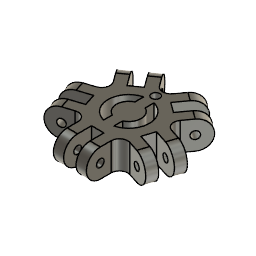
CenterRingV0_v10 (Autodesk Fusion 360 design; units mm, degrees)
Autodesk Fusion 360 part; units mm, degrees
sketch "Sketch1" plane through (0, 0, 0) normal (0, 0, 1) x (1, 0, 0)
  circle A0 centre (0, 0) radius 5
  circle A1 centre (0, 0) radius 7.5
  line L0 (0, 0) -> (0, -7.5) construction
  line L1 (0, -7.5) -> (1.5, -7.5) construction
  line L2 (0, -7.5) -> (-1.5, -7.5) construction
  line L3 (-1.5, -7.5) -> (-1.5, -7.3485)
  line L4 (1.5, -7.5) -> (1.5, -7.3485)
  line L5 (1.5, -7.5) -> (1.5, -14.25)
  line L6 (0, -7.5) -> (0, -9.25) construction
  line L7 (0, -9.25) -> (1.5, -9.25) construction
  line L8 (0, -9.25) -> (-1.5, -9.25) construction
  line L9 (0, -9.25) -> (0, -11.75) construction
  line L10 (1.5, -7.5) -> (-1.5, -7.5)
  line L11 (-1.5, -7.5) -> (-1.5, -14.25)
  line L12 (1.5, -14.25) -> (4, -14.25)
  line L13 (4, -14.25) -> (4, -6.3443)
  line L14 (-1.5, -14.25) -> (-4, -14.25)
  line L15 (-4, -14.25) -> (-4, -6.3443)
  dimension "d1" = 10
  dimension "d4" = 15
  dimension "d5" = 1.5
  dimension "d6" = 1.5
  dimension "d7" = 6.75
  dimension "d8" = 1.75
  dimension "d9" = 2.5
  dimension "d10" = 3
  dimension "d14" = 6.75
  constraint coincident A0.centre A1.centre
  constraint concentric A0 A1
  constraint coincident A1 L0.end
  constraint vertical L0
  constraint perpendicular L0 L1
  constraint perpendicular L0 L2
  constraint coincident A1 L3.end
  constraint perpendicular L2 L3
  constraint coincident A1 L4.end
  constraint perpendicular L1 L4
  constraint perpendicular L1 L5
  constraint coincident L5 L7.end
  constraint perpendicular L5 L7
  constraint perpendicular L7 L9
  constraint horizontal L10
  constraint vertical L11
  constraint perpendicular L5 L12
  constraint coincident A1 L13.end
  constraint perpendicular L12 L13
  constraint perpendicular L11 L14
  constraint coincident A1 L15.end
  constraint perpendicular L14 L15
  measures "d1" diameter of A0
  measures "d4" diameter of A1
  measures "d5" distance of L0.end L1.end
  measures "d6" distance of L0.end L2.end
  measures "d7" distance of L1.end L5.end
  measures "d8" distance of L0.end L6.end
  measures "d9" distance of L6.end L9.end
  measures "d10" distance of L1.end L2.end
  measures "d14" distance of L2.end L11.end
extrude "Extrude1" add sketch "Sketch1" along normal blind 6.75 makes body 1
sketch "Sketch2" plane through (-1.5, 0, 0) normal (1, 0, 0) x (0, 1, 0)
  line L0 (-14.25, 0) -> (-7.5, 0)
  line L1 (-7.5, 0) -> (-7.5, 6.75)
  line L2 (-7.5, 6.75) -> (-14.25, 6.75)
  line L3 (-14.25, 6.75) -> (-14.25, 0)
  line L4 (-14.25, 6.75) -> (-7.5, 6.75)
  line L5 (-7.5, 6.75) -> (-7.5, 0)
  line L6 (-7.5, 0) -> (-14.25, 0)
  line L7 (-14.25, 0) -> (-14.25, 6.75)
  line L8 (-14.25, 6.75) -> (-7.5, 0) construction
  circle A0 centre (-10.875, 3.375) radius 0.925
  circle A1 centre (-10.875, 3.375) radius 3.375
  dimension "d12" = 6.75
  dimension "d13" = 6.75
  dimension "d15" = 1.85
  constraint horizontal L4
  constraint vertical L5
  constraint horizontal L6
  constraint vertical L7
  constraint coincident L0.end L1.start
  constraint coincident L2.end L3.start
  constraint midpoint L8 A0.centre
  constraint concentric A0 A1
  constraint tangent L6 A1
  measures "d12" distance of L1.end L0.end
  measures "d13" distance of L2.end L1.end
  measures "d15" diameter of A0
extrude "Extrude2" cut sketch "Sketch2" along normal blind 14 and the other way blind 5 contours L0 L3 L6 L7 A1 | L2 L3 L4 L7 A1 | A0 bodies 1
pattern_circular "C-Pattern1" count 5 over 360 about axis through (0, 0, 1.75) along (0, 0, 1) of bodies 1 makes body 2 at (8.815, 0.4655, 0) makes body 3 at (7.4051, 4.8048, 0) makes body 4 at (-2.2813, 8.5274, 6.75) makes body 5 at (-6.8579, -5.5579, 0)
combine "Combine1" operation add target body 5 tool bodies 2 1 4 3
fillet "Fillet1" radius 2 10 edges at (4, -6.3443, 3.375) (4.7977, -5.7647, 3.375) (6.9651, 2.7815, 3.375) (7.2698, 1.8437, 3.375) (-0.493, 7.4838, 3.375) (0.493, 7.4838, 3.375) (-6.9651, 2.7815, 3.375) (-7.2698, 1.8437, 3.375) (-4.7977, -5.7647, 3.375) (-4, -6.3443, 3.375) on bodies 5
sketch "Sketch3" plane through (0, 0, 6.75) normal (0, 0, 1) x (-1, 0, 0)
  circle A0 centre (0, 0) radius 5
  arc A1 (-8.0902, -4.33) -> (-9.0902, -1.2523) centre (-9.7082, -3.1544) ccw
  line L0 (-8.0902, -4.33) -> (-9.6282, -6.4469)
  line L1 (-9.6282, -6.4469) -> (-7.6057, -7.9164)
  line L2 (-7.6057, -7.9164) -> (-5.6219, -5.1859)
  line L3 (-5.6219, -5.1859) -> (-3.1949, -6.9493)
  line L4 (-3.1949, -6.9493) -> (-5.1786, -9.6797)
  line L5 (-5.1786, -9.6797) -> (-3.1561, -11.1492)
  line L6 (-3.1561, -11.1492) -> (-1.618, -9.0322)
  arc A2 (1.618, -9.0322) -> (-1.618, -9.0322) centre (0, -10.2078) ccw
  line L7 (1.618, -9.0322) -> (3.1561, -11.1492)
  line L8 (3.1561, -11.1492) -> (5.1786, -9.6797)
  line L9 (5.1786, -9.6797) -> (3.1949, -6.9493)
  line L10 (3.1949, -6.9493) -> (5.6219, -5.1859)
  line L11 (5.6219, -5.1859) -> (7.6057, -7.9164)
  line L12 (7.6057, -7.9164) -> (9.6282, -6.4469)
  line L13 (9.6282, -6.4469) -> (8.0902, -4.33)
  arc A3 (9.0902, -1.2523) -> (8.0902, -4.33) centre (9.7082, -3.1544) ccw
  line L14 (9.0902, -1.2523) -> (11.5788, -0.4437)
  line L15 (11.5788, -0.4437) -> (10.8063, 1.934)
  line L16 (10.8063, 1.934) -> (7.5964, 0.891)
  line L17 (7.5964, 0.891) -> (6.6694, 3.7442)
  line L18 (6.6694, 3.7442) -> (9.8792, 4.7871)
  line L19 (9.8792, 4.7871) -> (9.1067, 7.1648)
  line L20 (9.1067, 7.1648) -> (6.618, 6.3562)
  arc A4 (4, 8.2583) -> (6.618, 6.3562) centre (6, 8.2583) ccw
  line L21 (4, 8.2583) -> (4, 10.875)
  line L22 (4, 10.875) -> (1.5, 10.875)
  line L23 (1.5, 10.875) -> (1.5, 7.5)
  line L24 (1.5, 7.5) -> (-1.5, 7.5)
  line L25 (-1.5, 7.5) -> (-1.5, 10.875)
  line L26 (-1.5, 10.875) -> (-4, 10.875)
  line L27 (-4, 10.875) -> (-4, 8.2583)
  arc A5 (-6.618, 6.3562) -> (-4, 8.2583) centre (-6, 8.2583) ccw
  line L28 (-6.618, 6.3562) -> (-9.1067, 7.1648)
  line L29 (-9.1067, 7.1648) -> (-9.8792, 4.7871)
  line L30 (-9.8792, 4.7871) -> (-6.6694, 3.7442)
  line L31 (-6.6694, 3.7442) -> (-7.5964, 0.891)
  line L32 (-7.5964, 0.891) -> (-10.8063, 1.934)
  line L33 (-10.8063, 1.934) -> (-11.5788, -0.4437)
  line L34 (-11.5788, -0.4437) -> (-9.0902, -1.2523)
  circle A6 centre (0, 0) radius 15
  circle A7 centre (0, 0) radius 5
  dimension "d24" = 30
  dimension "d25" = 10
  constraint concentric A0 A6
  constraint concentric A6 A7
  measures "d24" diameter of A6
  measures "d25" diameter of A7
sketch "Sketch4" plane through (0, 0, 6.75) normal (0, 0, 1) x (-1, 0, 0)
  circle A0 centre (0, 0) radius 5
  arc A1 (-8.0902, -4.33) -> (-9.0902, -1.2523) centre (-9.7082, -3.1544) ccw
  line L0 (-8.0902, -4.33) -> (-9.6282, -6.4469)
  line L1 (-9.6282, -6.4469) -> (-7.6057, -7.9164)
  line L2 (-7.6057, -7.9164) -> (-5.6219, -5.1859)
  line L3 (-5.6219, -5.1859) -> (-3.1949, -6.9493)
  line L4 (-3.1949, -6.9493) -> (-5.1786, -9.6797)
  line L5 (-5.1786, -9.6797) -> (-3.1561, -11.1492)
  line L6 (-3.1561, -11.1492) -> (-1.618, -9.0322)
  arc A2 (1.618, -9.0322) -> (-1.618, -9.0322) centre (0, -10.2078) ccw
  line L7 (1.618, -9.0322) -> (3.1561, -11.1492)
  line L8 (3.1561, -11.1492) -> (5.1786, -9.6797)
  line L9 (5.1786, -9.6797) -> (3.1949, -6.9493)
  line L10 (3.1949, -6.9493) -> (5.6219, -5.1859)
  line L11 (5.6219, -5.1859) -> (7.6057, -7.9164)
  line L12 (7.6057, -7.9164) -> (9.6282, -6.4469)
  line L13 (9.6282, -6.4469) -> (8.0902, -4.33)
  arc A3 (9.0902, -1.2523) -> (8.0902, -4.33) centre (9.7082, -3.1544) ccw
  line L14 (9.0902, -1.2523) -> (11.5788, -0.4437)
  line L15 (11.5788, -0.4437) -> (10.8063, 1.934)
  line L16 (10.8063, 1.934) -> (7.5964, 0.891)
  line L17 (7.5964, 0.891) -> (6.6694, 3.7442)
  line L18 (6.6694, 3.7442) -> (9.8792, 4.7871)
  line L19 (9.8792, 4.7871) -> (9.1067, 7.1648)
  line L20 (9.1067, 7.1648) -> (6.618, 6.3562)
  arc A4 (4, 8.2583) -> (6.618, 6.3562) centre (6, 8.2583) ccw
  line L21 (4, 8.2583) -> (4, 10.875)
  line L22 (4, 10.875) -> (1.5, 10.875)
  line L23 (1.5, 10.875) -> (1.5, 7.5)
  line L24 (1.5, 7.5) -> (-1.5, 7.5)
  line L25 (-1.5, 7.5) -> (-1.5, 10.875)
  line L26 (-1.5, 10.875) -> (-4, 10.875)
  line L27 (-4, 10.875) -> (-4, 8.2583)
  arc A5 (-6.618, 6.3562) -> (-4, 8.2583) centre (-6, 8.2583) ccw
  line L28 (-6.618, 6.3562) -> (-9.1067, 7.1648)
  line L29 (-9.1067, 7.1648) -> (-9.8792, 4.7871)
  line L30 (-9.8792, 4.7871) -> (-6.6694, 3.7442)
  line L31 (-6.6694, 3.7442) -> (-7.5964, 0.891)
  line L32 (-7.5964, 0.891) -> (-10.8063, 1.934)
  line L33 (-10.8063, 1.934) -> (-11.5788, -0.4437)
  line L34 (-11.5788, -0.4437) -> (-9.0902, -1.2523)
  circle A6 centre (0, 0) radius 3
  line L35 (1.25, 5.2869) -> (-1.25, 5.2869)
  line L36 (-1.25, 5.2869) -> (-1.25, -5.2869)
  line L37 (-1.25, -5.2869) -> (1.25, -5.2869)
  line L38 (1.25, -5.2869) -> (1.25, 5.2869)
  line L39 (1.25, 5.2869) -> (-1.25, -5.2869) construction
  line L40 (-1.25, 5.2869) -> (1.25, -5.2869) construction
  dimension "d31" = 6
  dimension "d32" = 2.5
  constraint coincident A0.centre A6.centre
  constraint horizontal L35
  constraint perpendicular L35 L36
  constraint parallel L35 L37
  constraint parallel L36 L38
  constraint coincident L39 A0.centre
  constraint coincident L40 A0.centre
  measures "d31" diameter of A6
  measures "d32" distance of L36.end L37.end
extrude "Extrude3" add sketch "Sketch4" against normal blind 6.75 contours A0 A6 L36 L38 | A0 A6 L36 L38 | A6 L36 L38 | A6 L38 | A6 L36 bodies 5
sketch "Sketch5" plane through (0, 0, 0) normal (0, 0, -1) x (1, 0, 0)
  arc A0 (-6.618, 6.3562) -> (-4, 8.2583) centre (-6, 8.2583) ccw
  line L0 (-6.618, 6.3562) -> (-9.1067, 7.1648)
  line L1 (-9.1067, 7.1648) -> (-9.8792, 4.7871)
  line L2 (-9.8792, 4.7871) -> (-6.6694, 3.7442)
  line L3 (-6.6694, 3.7442) -> (-7.5964, 0.891)
  line L4 (-7.5964, 0.891) -> (-10.8063, 1.934)
  line L5 (-10.8063, 1.934) -> (-11.5788, -0.4437)
  line L6 (-11.5788, -0.4437) -> (-9.0902, -1.2523)
  arc A1 (-8.0902, -4.33) -> (-9.0902, -1.2523) centre (-9.7082, -3.1544) ccw
  line L7 (-8.0902, -4.33) -> (-9.6282, -6.4469)
  line L8 (-9.6282, -6.4469) -> (-7.6057, -7.9164)
  line L9 (-7.6057, -7.9164) -> (-5.6219, -5.1859)
  line L10 (-5.6219, -5.1859) -> (-3.1949, -6.9493)
  line L11 (-3.1949, -6.9493) -> (-5.1786, -9.6797)
  line L12 (-5.1786, -9.6797) -> (-3.1561, -11.1492)
  line L13 (-3.1561, -11.1492) -> (-1.618, -9.0322)
  arc A2 (1.618, -9.0322) -> (-1.618, -9.0322) centre (0, -10.2078) ccw
  line L14 (1.618, -9.0322) -> (3.1561, -11.1492)
  line L15 (3.1561, -11.1492) -> (5.1786, -9.6797)
  line L16 (5.1786, -9.6797) -> (3.1949, -6.9493)
  line L17 (3.1949, -6.9493) -> (5.6219, -5.1859)
  line L18 (5.6219, -5.1859) -> (7.6057, -7.9164)
  line L19 (7.6057, -7.9164) -> (9.6282, -6.4469)
  line L20 (9.6282, -6.4469) -> (8.0902, -4.33)
  arc A3 (9.0902, -1.2523) -> (8.0902, -4.33) centre (9.7082, -3.1544) ccw
  line L21 (9.0902, -1.2523) -> (11.5788, -0.4437)
  line L22 (11.5788, -0.4437) -> (10.8063, 1.934)
  line L23 (10.8063, 1.934) -> (7.5964, 0.891)
  line L24 (7.5964, 0.891) -> (6.6694, 3.7442)
  line L25 (6.6694, 3.7442) -> (9.8792, 4.7871)
  line L26 (9.8792, 4.7871) -> (9.1067, 7.1648)
  line L27 (9.1067, 7.1648) -> (6.618, 6.3562)
  arc A4 (4, 8.2583) -> (6.618, 6.3562) centre (6, 8.2583) ccw
  line L28 (4, 8.2583) -> (4, 10.875)
  line L29 (4, 10.875) -> (1.5, 10.875)
  line L30 (1.5, 10.875) -> (1.5, 7.5)
  line L31 (1.5, 7.5) -> (-1.5, 7.5)
  line L32 (-1.5, 7.5) -> (-1.5, 10.875)
  line L33 (-1.5, 10.875) -> (-4, 10.875)
  line L34 (-4, 10.875) -> (-4, 8.2583)
  arc A5 (1.25, -4.8412) -> (1.25, 4.8412) centre (0, 0) ccw
  circle A6 centre (0, -6.5) radius 1
  line L35 (1.25, -4.8412) -> (1.25, -2.7272)
  line L36 (-1.25, 4.8412) -> (-1.25, 2.7272)
  arc A7 (1.25, -2.7272) -> (1.25, 2.7272) centre (0, 0) ccw
  line L37 (1.25, 2.7272) -> (1.25, 4.8412)
  arc A8 (-1.25, 2.7272) -> (-1.25, -2.7272) centre (0, 0) ccw
  line L38 (-1.25, -2.7272) -> (-1.25, -4.8412)
  arc A9 (-1.25, 4.8412) -> (-1.25, -4.8412) centre (0, 0) ccw
  dimension "d33" = 2
  measures "d33" diameter of A6
extrude "Extrude5" cut sketch "Sketch5" against normal blind 14 contours A6 bodies 5
